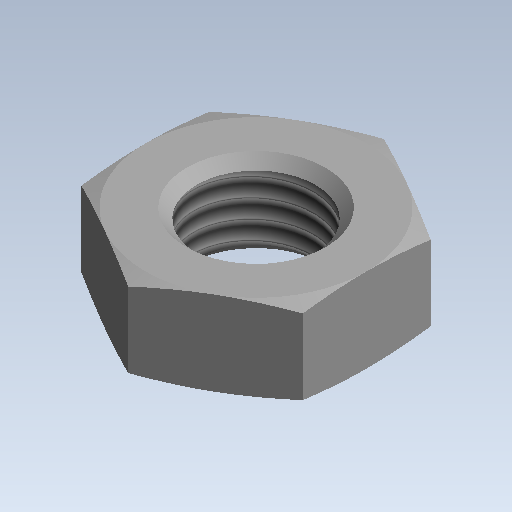
# Autodesk Inventor part: D-746
Saved by Autodesk Inventor 2020 (Build 240168000, 168)
## iProperties
Part Number: D-746
Material: Generic
Catalog Web Link: www.cadenas.de
Description: Mounting Nut for Original Line Cylinders-
Vendor: BIMBA
Document SubType Name: Modeling
Designer: partserver
Manufacturer: BIMBA
Mass: 0.489793 g
Surface Area: 5.017 cm^2
Volume: 0.489793 cm^3
Density: 1 g/cm^3
Appearance: PSOLRGB-191-191-191
Category: PARTsolutions
Company: BIMBA
PSOL_IDENT_0: {$CADENAS_DATA\23d-libs\bimba\bimba_brand\bimba_imperial\bimba_full_line\original_line_cylinders\acc
PSOL_IDENT_1: essories\mounting_nut.prj},188 {VTYP=3D},{NB=D-746},{LINA=D-746},{NN=Mounting Nut for Original Line
PSOL_IDENT_2: Cylinders},{DATE=19.01.2022 10:19:28},{GEOMDATE=10.11.2011 00:00:00},{VERSION=},{LINEID=240},{WBVAR=
PSOL_IDENT_3: MAT},{WBNUMERIC=}  {NB=D-746},{LINA=D-746},{KT=DUMMY},{PN=D-746},{PN1=D-746},{C=5/16-24},{TH=UNF},{M
PSOL_IDENT_4: AT=},{MAT1='','Zinc-Plated Carbon Steel', '-SS', 'Stainless Steel'},{A=0.50},{A1=0.50000000},{B=0.19
PSOL_IDENT_5: },{B1=0.19000000},{NDM=0.31250000},{PITCH=0.0417},{DIA=-},{DIA2=-},{DIA3=-},{DIA1=0},{DIA4=0.0000000
PSOL_IDENT_6: 0},{DIA5=0.00000000},{T=-},{T2=-},{T3=-},{T1=0},{T4=0.00000000},{T5=0.00000000},{COLOR=0.75,0.75,0.7
PSOL_IDENT_7: 5,0.00},{TT=0.05000000},{TO=0.20000000},{PRA=1}
NB: D-746
NN: Mounting Nut for Original Line Cylinders
NBSYN: $PN.
LINA: D-746
CATALOG: Bimba Products
PN: D-746
C: 5/16-24
MAT: Zinc-Plated Carbon Steel
A: 0.5
B: 0.19
DIA: -
T: -
SUPPLIER: BIMBA
ARTICLENO: D-746
BOMINFO: D-746
CREATOR: CADENAS GmbH
Title: D-746
Author: Cadenas PARTsolutions
Autodesk Inventor part; units mm, degrees
sketch "Sketch_8" plane through (0, 0, 0) normal (1, 0, 0) x (0, 1, 0)
  line L0 (0, -4.826) -> (0, 0)
  line L1 (0, 0) -> (6.35, 0)
  line L2 (6.35, 0) -> (7.62, -0.3403)
  line L3 (7.62, -0.3403) -> (7.62, -4.4857)
  line L4 (7.62, -4.4857) -> (6.35, -4.826)
  line L5 (6.35, -4.826) -> (0, -4.826)
  line L6 (0, -4.826) -> (0, 0)
  constraints: 14 end point
sketch "Sketch_10" plane through (0, 0, 0) normal (0, 0, 1) x (1, 0, 0)
  line L0 (-12.7, -12.7) -> (12.7, -12.7)
  line L1 (12.7, -12.7) -> (12.7, 12.7)
  line L2 (12.7, 12.7) -> (-12.7, 12.7)
  line L3 (-12.7, 12.7) -> (-12.7, -12.7)
  line L4 (-6.35, -3.6662) -> (0, -7.3323)
  line L5 (0, -7.3323) -> (6.35, -3.6662)
  line L6 (6.35, -3.6662) -> (6.35, 3.6662)
  line L7 (6.35, 3.6662) -> (0, 7.3323)
  line L8 (0, 7.3323) -> (-6.35, 3.6662)
  line L9 (-6.35, 3.6662) -> (-6.35, -3.6662)
  constraints: 20 end point
revolve "Revolution1" add sketch "Sketch_8" angle 360 about axis through (0, 0, -4.826) along (0, 0, -1)
extrude "Extrusion1" cut sketch "Sketch_10" against normal blind 4.826
sketch "Sketch_11" plane through (0, 0, 0) normal (1, 0, 0) x (0, 1, 0)
  line L0 (0, -4.826) -> (0, 0)
  line L1 (0, 0) -> (3.9688, 0)
  line L2 (3.9688, 0) -> (3.396, -0.5728)
  line L3 (3.396, -0.5728) -> (3.396, -4.2532)
  line L4 (3.396, -4.2532) -> (3.9688, -4.826)
  line L5 (3.9688, -4.826) -> (0, -4.826)
  line L6 (0, -4.826) -> (0, 0)
  constraints: 14 end point
revolve "Revolution2" cut sketch "Sketch_11" angle 360 about axis through (0, 0, -4.826) along (0, 0, -1)
thread "Thread1" size "5/16-24 UNF" class "2B" standard "ANSI Unified Screw Threads" full length
ref_plane "NUT_XY" through (0, 0, 0) normal (0, 0, 1) x (1, 0, 0)
ref_plane "NUT_YZ" through (0, 0, 0) normal (1, 0, 0) x (0, 1, 0)
ref_plane "NUT_ZX" through (0, 0, 0) normal (0, 1, 0) x (0, 0, 1)
ref_plane "a1_XY" through (-6.35, 6.35, 0) normal (0, 0, 1) x (1, 0, 0)
ref_plane "a1_YZ" through (-6.35, 6.35, 0) normal (1, 0, 0) x (0, 1, 0)
ref_plane "a1_ZX" through (-6.35, 6.35, 0) normal (0, 1, 0) x (0, 0, 1)
ref_plane "a2_XY" through (6.35, 6.35, 0) normal (0, 0, 1) x (1, 0, 0)
ref_plane "a2_YZ" through (6.35, 6.35, 0) normal (1, 0, 0) x (0, 1, 0)
ref_plane "a2_ZX" through (6.35, 6.35, 0) normal (0, 1, 0) x (0, 0, 1)
ref_plane "b1_XY" through (0, 6.35, 0) normal (1, 0, 0) x (0, 0, -1)
ref_plane "b1_YZ" through (0, 6.35, 0) normal (0, 0, -1) x (0, 1, 0)
ref_plane "b1_ZX" through (0, 6.35, 0) normal (0, 1, 0) x (1, 0, 0)
ref_plane "b2_XY" through (0, 6.35, -4.826) normal (1, 0, 0) x (0, 0, -1)
ref_plane "b2_YZ" through (0, 6.35, -4.826) normal (0, 0, -1) x (0, 1, 0)
ref_plane "b2_ZX" through (0, 6.35, -4.826) normal (0, 1, 0) x (1, 0, 0)
ref_plane "e_XY" through (0, 0, -4.826) normal (1, 0, 0) x (0, 0, -1)
ref_plane "e_YZ" through (0, 0, -4.826) normal (0, 0, -1) x (0, 1, 0)
ref_plane "e_ZX" through (0, 0, -4.826) normal (0, 1, 0) x (1, 0, 0)
ref_plane "ol1_XY" through (0, 0, -6.35) normal (0, 1, 0) x (1, 0, 0)
ref_plane "ol1_YZ" through (0, 0, -6.35) normal (1, 0, 0) x (0, 0, -1)
ref_plane "ol1_ZX" through (0, 0, -6.35) normal (0, 0, -1) x (0, 1, 0)
ref_plane "ol2_XY" through (4.826, 0, -6.35) normal (0, 1, 0) x (1, 0, 0)
ref_plane "ol2_YZ" through (4.826, 0, -6.35) normal (1, 0, 0) x (0, 0, -1)
ref_plane "ol2_ZX" through (4.826, 0, -6.35) normal (0, 0, -1) x (0, 1, 0)
ref_plane "th1_XY" through (0, 3.9688, -4.826) normal (1, 0, 0) x (0, 0, -1)
ref_plane "th1_YZ" through (0, 3.9688, -4.826) normal (0, 0, -1) x (0, 1, 0)
ref_plane "th1_ZX" through (0, 3.9688, -4.826) normal (0, 1, 0) x (1, 0, 0)
ref_plane "th2_XY" through (0, -3.9688, -4.826) normal (1, 0, 0) x (0, 0, -1)
ref_plane "th2_YZ" through (0, -3.9688, -4.826) normal (0, 0, -1) x (0, 1, 0)
ref_plane "th2_ZX" through (0, -3.9688, -4.826) normal (0, 1, 0) x (1, 0, 0)
body "Solid1"
